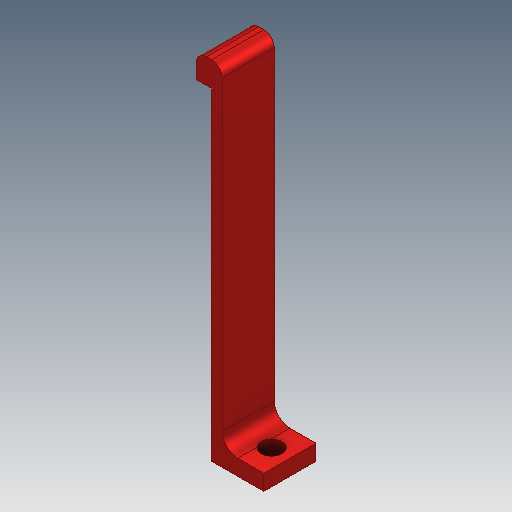
# Autodesk Inventor part: vacuum_bin_holder
Saved by Autodesk Inventor 2020 (Build 240168000, 168)
## iProperties
Created: 2022-08-13
Part Number: vacuum_bin_holder
Material: Aluminum, Anodized Red
Document SubType Name: Modeling
Designer: Umair
Density: 2.7 g/cm^3
Appearance: Anodized - Red
Author: Umair
Autodesk Inventor part; units mm, degrees
ref_plane "YZ Plane" through (0, 0, 0) normal (1, 0, 0) x (0, 1, 0)
ref_plane "XZ Plane" through (0, 0, 0) normal (0, 1, 0) x (-1, 0, 0)
ref_plane "XY Plane" through (0, 0, 0) normal (0, 0, 1) x (1, 0, 0)
sketch "Sketch1" plane through (0, 0, 0) normal (0, 1, 0) x (-1, 0, 0)
  line L0 (0, 0) -> (-10, 0)
  line L1 (-10, 0) -> (-10, -10)
  line L2 (-10, -10) -> (0, -10)
  line L3 (0, -10) -> (0, 0)
  line L4 (0, 0) -> (-2, 0)
  line L5 (-2, 0) -> (-2, -10)
  dimension "d0" = 10
  dimension "d1" = 10
  dimension "d2" = 2
  constraints: 12 end point, 4 perpendicular, 2 point on line, 1 horizontal
  measures "d0" distance of L0.start L0.end
  measures "d1" distance of L0.end L1.end
  measures "d2" distance of L0.start L4.end
extrude "Extrusion1" add sketch "Sketch1" along normal blind 3 contours L5 L2 L1 L0
extrude "Extrusion2" add sketch "Sketch1" along normal blind 62 contours L3 L2 L5 L0
sketch "Sketch2" plane through (0, 3, 0) normal (0, 1, 0) x (1, 0, 0)
  line L0 (9.919, 10.0415) -> (10, 5)
  line L1 (10, 0) -> (10, 10) projected
  line L2 (10, 5) -> (6.5, 5)
  line L3 (2, 0) -> (2, 10) projected
  circle A0 centre (6.5, 5) radius 2
  point P0 (0, 0)
  dimension "d7" = 3.5
  dimension "d8" = 4
  constraints: 4 end point, 1 centre point, 1 coincident, 1 midpoint, 1 perpendicular
  measures "d7" distance of L0.end L2.end
  measures "d8" diameter of A0
extrude "Extrusion3" cut sketch "Sketch2" against normal blind 62
fillet "Fillet1" radius 3 1 edges at (2, 3, -5)
sketch "Sketch3" plane through (0, 0, -10) normal (-1, 0, 0) x (0, 0, 1)
  line L0 (0, 0) -> (0, 62) projected
  line L1 (0, 62) -> (0, 66.7685)
  line L2 (0, 66.7685) -> (10, 66.7685)
  line L3 (10, 66.7685) -> (10, 62)
  line L4 (10, 62) -> (0, 62) projected
  line L5 (10, 62) -> (0, 62)
  point P0 (10, 0)
  constraints: 8 end point, 2 perpendicular, 1 collinear, 1 vertical
extrude "Extrusion4" add sketch "Sketch3" along normal blind 3 and the other way blind 2
fillet "Fillet2" radius 2 2 edges at (2, 66.7685, -5) (-3, 66.7685, -5)
body "Solid1"
